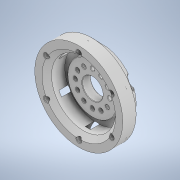
# Autodesk Inventor part: TopFlywheelClamp2
Saved by Autodesk Inventor 2020 (Build 240168000, 168)
## iProperties
Created: 2020-02-07
Part Number: TopFlywheelClamp2
Material: Generic
Document SubType Name: Modeling
Designer: srini
Density: 1 g/cm^3
Appearance: Default
Author: srini
Autodesk Inventor part; units mm, degrees
ref_plane "YZ Plane" through (0, 0, 0) normal (1, 0, 0) x (0, 1, 0)
ref_plane "XZ Plane" through (0, 0, 0) normal (0, 1, 0) x (-1, 0, 0)
sketch "Sketch1" plane through (0, 0, 0) normal (0, 0, 1) x (1, 0, 0)
  circle A0 centre (0, 0) radius 61.2775
  dimension "d0" = 122.555
  constraints: 1 centre point, 1 coincident
  measures "d0" diameter of A0
extrude "Extrusion1" add sketch "Sketch1" along normal blind 31.242
sketch "Sketch2" plane through (0, 0, 31.242) normal (0, 0, 1) x (1, 0, 0)
  circle A0 centre (0, 0) radius 44.577
  circle A1 centre (0, 0) radius 34.798
  dimension "d3" = 69.596
  dimension "d4" = 89.154
  constraints: 2 centre point, 2 coincident
  measures "d3" diameter of A1
  measures "d4" diameter of A0
extrude "Extrusion2" cut sketch "Sketch2" against normal blind 25.146
sketch "Sketch3" plane through (0, 0, 31.242) normal (0, 0, 1) x (1, 0, 0)
  circle A0 centre (0, 0) radius 34.798 projected
extrude "Extrusion3" cut sketch "Sketch3" against normal blind 19.05
chamfer "Chamfer1" distance 12.7 angle 45 1 edges at (-61.2775, 0, 0)
ref_plane "Work Plane1" through (0, 0, 18.542) normal (0, 0, 1) x (1, 0, 0)
sketch "Sketch5" plane through (0, 0, 18.542) normal (0, 0, 1) x (1, 0, 0)
  circle A0 centre (0, 52.3875) radius 3.373438
  circle A1 centre (-45.368906, 26.19375) radius 3.373438
  circle A2 centre (-45.368906, -26.19375) radius 3.373438
  circle A3 centre (0, -52.3875) radius 3.373438
  circle A4 centre (45.368906, -26.19375) radius 3.373438
  circle A5 centre (45.368906, 26.19375) radius 3.373438
  point P0 (0, 0)
  dimension "d13" = 52.3875
  dimension "d16" = 360
  dimension "d18" = 6.74688
  constraints: 6 centre point, 1 vertical alignment, 13 other
  measures "d13" distance of A0.centre point (0, 0)
  measures "d18" diameter of A0
extrude "Extrusion4" cut sketch "Sketch5" against normal through all both and the other way through all
sketch "Sketch6" plane through (0, 0, 18.542) normal (0, 0, 1) x (1, 0, 0)
  circle A0 centre (-45.368906, -26.19375) radius 3.373438
  circle A1 centre (-45.368906, -26.19375) radius 8.763
  circle A2 centre (0, -52.3875) radius 8.763
  circle A3 centre (45.368906, -26.19375) radius 8.763
  circle A4 centre (45.368906, 26.19375) radius 8.763
  circle A5 centre (0, 52.3875) radius 8.763
  circle A6 centre (-45.368906, 26.19375) radius 8.763
  point P0 (0, 0)
  dimension "d28" = 17.526
  dimension "d31" = 360
  constraints: 6 centre point, 1 coincident, 13 other
  measures "d28" diameter of A1
extrude "Extrusion5" cut sketch "Sketch6" against normal through all contours A0 | A1 | A2 | A3 | A4 | A5 | A6
sketch "Sketch8" plane through (0, 0, 0) normal (0, 0, -1) x (-1, 0, 0)
  circle A0 centre (0, 0) radius 14.3002
  circle A1 centre (0, -23.8125) radius 2.579688
  circle A2 centre (11.90625, -20.62223) radius 2.579688
  circle A3 centre (20.62223, -11.90625) radius 2.579688
  circle A4 centre (23.8125, 0) radius 2.579688
  circle A5 centre (20.62223, 11.90625) radius 2.579688
  circle A6 centre (11.90625, 20.62223) radius 2.579688
  circle A7 centre (0, 23.8125) radius 2.579688
  circle A8 centre (-11.90625, 20.62223) radius 2.579688
  circle A9 centre (-20.62223, 11.90625) radius 2.579688
  circle A10 centre (-23.8125, 0) radius 2.579688
  circle A11 centre (-20.62223, -11.90625) radius 2.579688
  circle A12 centre (-11.90625, -20.62223) radius 2.579688
  dimension "d33" = 28.6004
  dimension "d34" = 5.15938
  dimension "d35" = 23.8125
  dimension "d38" = 360
  constraints: 13 centre point, 1 coincident, 1 vertical alignment, 25 other
  measures "d33" diameter of A0
  measures "d34" diameter of A1
  measures "d35" distance of point (0, 0) A1.centre
extrude "Extrusion6" cut sketch "Sketch8" against normal through all
chamfer "Chamfer2" distance 0.635 angle 45 33 edges at (14.3002, 0, 0) (2.5797, -23.8125, 0) (-9.3266, -20.6222, 0) (-18.0425, -11.9063, 0) (-21.2328, 0, 0) (-18.0425, 11.9062, 0) (-9.3266, 20.6222, 0) (2.5797, 23.8125, 0) (14.4859, 20.6222, 0) (23.2019, 11.9063, 0) (26.3922, 0, 0) (23.2019, -11.9062, 0) (14.4859, -20.6222, 0) (-34.798, 0, 12.192) (-48.7423, 26.1938, 31.242) (-3.3734, 52.3875, 31.242) (41.9955, 26.1937, 31.242) (41.9955, -26.1938, 31.242) (-3.3734, -52.3875, 31.242) (-48.7423, -26.1938, 31.242) (2.5797, 23.8125, 12.192) (-9.3266, 20.6222, 12.192) (-18.0425, 11.9062, 12.192) (-21.2328, 0, 12.192) (-18.0425, -11.9063, 12.192) (-9.3266, -20.6222, 12.192) (2.5797, -23.8125, 12.192) (14.4859, -20.6222, 12.192) (23.2019, -11.9062, 12.192) (26.3922, 0, 12.192) (23.2019, 11.9063, 12.192) (14.4859, 20.6222, 12.192) (14.3002, 0, 12.192)
sketch "Sketch9" plane through (0, 0, 18.542) normal (0, 0, -1) x (-1, 0, 0)
  line L0 (46.828923, -16.918051) -> (38.065923, -32.096012)
  line L1 (38.065923, -32.096012) -> (43.908888, -35.469449)
  line L2 (43.908888, -35.469449) -> (52.671888, -20.291488)
  line L3 (52.671888, -20.291488) -> (46.828923, -16.918051)
  circle A0 centre (45.368906, -26.19375) radius 3.373438
  line L4 (46.828923, -16.918051) -> (43.908888, -35.469449) construction
  line L5 (38.065923, -32.096012) -> (52.671888, -20.291488) construction
  line L6 (48.290388, -27.880469) -> (42.447423, -24.507031) construction
  circle A1 centre (45.368906, -26.19375) radius 3.373438
  line L7 (38.065923, 32.096012) -> (46.828923, 16.918051)
  line L8 (46.828923, 16.918051) -> (52.671888, 20.291488)
  line L9 (52.671888, 20.291488) -> (43.908888, 35.469449)
  line L10 (43.908888, 35.469449) -> (38.065923, 32.096012)
  line L11 (38.065923, 32.096012) -> (52.671888, 20.291488) construction
  line L12 (46.828923, 16.918051) -> (43.908888, 35.469449) construction
  line L13 (48.290388, 27.880469) -> (42.447423, 24.507031) construction
  line L14 (-8.763, 49.014063) -> (8.763, 49.014063)
  line L15 (8.763, 49.014063) -> (8.763, 55.760938)
  line L16 (8.763, 55.760938) -> (-8.763, 55.760938)
  line L17 (-8.763, 55.760938) -> (-8.763, 49.014063)
  line L18 (-8.763, 49.014063) -> (8.763, 55.760938) construction
  line L19 (8.763, 49.014063) -> (-8.763, 55.760938) construction
  line L20 (0, 55.760937) -> (0, 49.014063) construction
  line L21 (-46.828923, 16.918051) -> (-38.065923, 32.096012)
  line L22 (-38.065923, 32.096012) -> (-43.908888, 35.469449)
  line L23 (-43.908888, 35.469449) -> (-52.671888, 20.291488)
  line L24 (-52.671888, 20.291488) -> (-46.828923, 16.918051)
  line L25 (-46.828923, 16.918051) -> (-43.908888, 35.469449) construction
  line L26 (-38.065923, 32.096012) -> (-52.671888, 20.291488) construction
  line L27 (-48.290388, 27.880469) -> (-42.447423, 24.507031) construction
  line L28 (-38.065923, -32.096012) -> (-46.828923, -16.918051)
  line L29 (-46.828923, -16.918051) -> (-52.671888, -20.291488)
  line L30 (-52.671888, -20.291488) -> (-43.908888, -35.469449)
  line L31 (-43.908888, -35.469449) -> (-38.065923, -32.096012)
  line L32 (-38.065923, -32.096012) -> (-52.671888, -20.291488) construction
  line L33 (-46.828923, -16.918051) -> (-43.908888, -35.469449) construction
  line L34 (-48.290388, -27.880469) -> (-42.447423, -24.507031) construction
  line L35 (8.763, -49.014063) -> (-8.763, -49.014063)
  line L36 (-8.763, -49.014063) -> (-8.763, -55.760938)
  line L37 (-8.763, -55.760938) -> (8.763, -55.760938)
  line L38 (8.763, -55.760938) -> (8.763, -49.014063)
  line L39 (8.763, -49.014063) -> (-8.763, -55.760938) construction
  line L40 (-8.763, -49.014063) -> (8.763, -55.760938) construction
  line L41 (0, -55.760938) -> (0, -49.014063) construction
  point P0 (0, 0)
  point P1 (0, 0)
  point P2 (0, 0)
  point P3 (0, 0)
  point P4 (0, 0)
  point P5 (0, 0)
  point P6 (44.246563, -34.884579)
  point P7 (52.334214, -20.876358)
  dimension "d47" = 360
  constraints: 84 end point, 6 point on line, 4 midpoint, 2 coincident, 2 parallel, 1 perpendicular, 1 tangent, 85 other
extrude "Extrusion7" cut sketch "Sketch9" against normal blind 0.3
sketch "Sketch10" plane through (0, 0, 18.842) normal (0, 0, -1) x (-1, 0, 0)
  line L0 (44.134142, -21.585549) -> (40.760705, -27.428514)
  line L1 (40.760705, -27.428514) -> (46.60367, -30.801951)
  line L2 (46.60367, -30.801951) -> (49.977107, -24.958986)
  line L3 (49.977107, -24.958986) -> (44.134142, -21.585549)
  circle A0 centre (45.368906, -26.19375) radius 4.008438 construction
  line L4 (44.134142, -21.585549) -> (46.60367, -30.801951) construction
  line L5 (40.760705, -27.428514) -> (49.977107, -24.958986) construction
  line L6 (48.290388, -27.880469) -> (42.447423, -24.507031) construction
  arc A1 (42.447423, -24.507031) -> (48.290388, -27.880469) centre (45.368906, -26.19375) ccw
  line L7 (40.760705, 27.428514) -> (44.134142, 21.585549)
  line L8 (44.134142, 21.585549) -> (49.977107, 24.958986)
  line L9 (49.977107, 24.958986) -> (46.60367, 30.801951)
  line L10 (46.60367, 30.801951) -> (40.760705, 27.428514)
  line L11 (40.760705, 27.428514) -> (49.977107, 24.958986) construction
  line L12 (44.134142, 21.585549) -> (46.60367, 30.801951) construction
  line L13 (48.290388, 27.880469) -> (42.447423, 24.507031) construction
  line L14 (-3.373437, 49.014063) -> (3.373438, 49.014063)
  line L15 (3.373438, 49.014063) -> (3.373438, 55.760938)
  line L16 (3.373438, 55.760938) -> (-3.373437, 55.760938)
  line L17 (-3.373437, 55.760938) -> (-3.373437, 49.014063)
  line L18 (-3.373437, 49.014063) -> (3.373438, 55.760938) construction
  line L19 (3.373438, 49.014063) -> (-3.373437, 55.760938) construction
  line L20 (0, 55.760938) -> (0, 49.014063) construction
  line L21 (-44.134142, 21.585549) -> (-40.760705, 27.428514)
  line L22 (-40.760705, 27.428514) -> (-46.60367, 30.801951)
  line L23 (-46.60367, 30.801951) -> (-49.977107, 24.958986)
  line L24 (-49.977107, 24.958986) -> (-44.134142, 21.585549)
  line L25 (-44.134142, 21.585549) -> (-46.60367, 30.801951) construction
  line L26 (-40.760705, 27.428514) -> (-49.977107, 24.958986) construction
  line L27 (-48.290388, 27.880469) -> (-42.447423, 24.507031) construction
  line L28 (-40.760705, -27.428514) -> (-44.134142, -21.585549)
  line L29 (-44.134142, -21.585549) -> (-49.977107, -24.958986)
  line L30 (-49.977107, -24.958986) -> (-46.60367, -30.801951)
  line L31 (-46.60367, -30.801951) -> (-40.760705, -27.428514)
  line L32 (-40.760705, -27.428514) -> (-49.977107, -24.958986) construction
  line L33 (-44.134142, -21.585549) -> (-46.60367, -30.801951) construction
  line L34 (-48.290388, -27.880469) -> (-42.447423, -24.507031) construction
  line L35 (3.373437, -49.014063) -> (-3.373438, -49.014063)
  line L36 (-3.373438, -49.014063) -> (-3.373438, -55.760938)
  line L37 (-3.373438, -55.760938) -> (3.373437, -55.760938)
  line L38 (3.373437, -55.760938) -> (3.373437, -49.014063)
  line L39 (3.373437, -49.014063) -> (-3.373438, -55.760938) construction
  line L40 (-3.373438, -49.014063) -> (3.373437, -55.760938) construction
  line L41 (0, -55.760938) -> (0, -49.014063) construction
  point P0 (0, 0)
  point P1 (0, 0)
  point P2 (42.447423, 24.507031)
  point P3 (48.290388, 27.880469)
  point P4 (0, 0)
  point P5 (0, 49.014063)
  point P6 (0, 55.760938)
  point P7 (0, 0)
  point P8 (-42.447423, 24.507031)
  point P9 (-48.290388, 27.880469)
  point P10 (0, 0)
  point P11 (-42.447423, -24.507031)
  point P12 (-48.290388, -27.880469)
  point P13 (0, 0)
  point P14 (0, -49.014063)
  point P15 (0, -55.760938)
  dimension "d53" = 360
  constraints: 84 end point, 6 point on line, 4 midpoint, 2 coincident, 2 parallel, 2 tangent, 1 perpendicular, 95 other
extrude "Extrusion8" cut sketch "Sketch10" against normal blind 0.3
chamfer "Chamfer3" distance 6.604 angle 45 1 edges at (-44.577, 0, 31.242)
body "Solid1"
